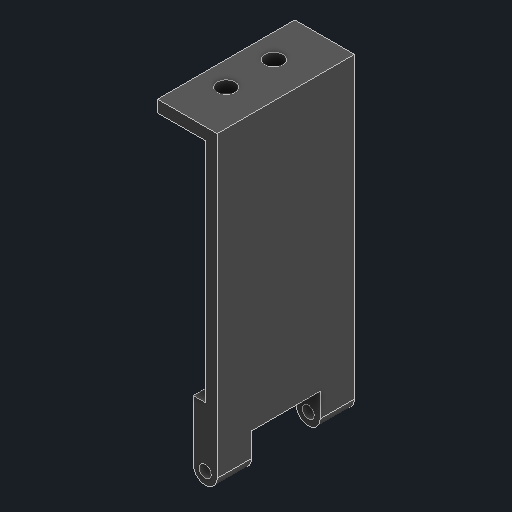
# Autodesk Inventor part: rudder_base
Saved by Autodesk Inventor 2024 (Build 280153000, 153)
## iProperties
Created: 2022-03-30
Part Number: rudder_base
Material: Generic
Document SubType Name: Modeling
Designer: kardo
Density: 1 g/cm^3
Appearance: Dark Plastic
Author: kardo
Autodesk Inventor part; units mm, degrees
ref_plane "YZ Plane" through (0, 0, 0) normal (1, 0, 0) x (0, 1, 0)
ref_plane "XZ Plane" through (0, 0, 0) normal (0, 1, 0) x (-1, 0, 0)
ref_plane "XY Plane" through (0, 0, 0) normal (0, 0, 1) x (1, 0, 0)
derived "parameters_powertrain.ipt"
sketch "sk_base" plane through (0, 0, 0) normal (0, 1, 0) x (-1, 0, 0)
  line L0 (16.1, 0) -> (-16.1, 0) construction
  line L1 (0, -4.6) -> (0, 27.6) construction
  line L2 (0, 23) -> (0, 15.5) construction
  line L3 (0, 7.5) -> (0, 0) construction
  dimension "d13" = 8
  dimension "d36" = 23
  constraints: 4 end point, 3 point on line, 1 collinear
  measures "d13" distance of L3.start L2.end
  measures "d36" distance from line of L0 L2.start
sketch "sk_length" plane through (0, 0, 0) normal (0, 0, 1) x (1, 0, 0)
  line L0 (0, -62.4) -> (0, 10.4) construction
  line L1 (-6, 0) -> (8, 0) construction
  arc A0 (2, -50) -> (6, -50) centre (4, -50) ccw
  line L2 (2, -50) -> (2, -40)
  line L3 (2, -40) -> (4, -40)
  line L4 (4, -40) -> (4, -2)
  line L5 (4, -2) -> (-4, -2)
  line L6 (-4, -2) -> (-4, 0)
  line L7 (-4, 0) -> (6, 0)
  line L8 (6, 0) -> (6, -50)
  point P0 (0, 0)
  dimension "d2" = 50
  dimension "d9" = 2
  dimension "d10" = 4
  dimension "d32" = 4
  dimension "d33" = 10
  dimension "d35" = 4
  constraints: 15 end point, 6 parallel, 3 point on line, 2 point on circle, 2 tangent, 1 centre point, 1 coincident
  measures "d2" distance from line of L1 A0.centre
  measures "d9" distance between parallel lines of L1 L5
  measures "d10" distance between parallel lines of L0 L6
  measures "d32" distance from line of L0 point (4, -50)
  measures "d33" distance of L2.start L2.end
  measures "d35" diameter of A0
extrude "extrude" add sketch "sk_length" along normal up to surface (23 mm away)
hole "drill_base" at (0, 0, 7.5) at (0, 0, 15.5) direction (0, -1, 0) diameter 3 depth 2 tip angle 118
sketch "sk_remove_fin_attach" plane through (2, -50, 0) normal (-1, 0, 0) x (0, 0, 1)
  line L0 (0, 10) -> (23, 10) projected
  line L1 (0, -2) -> (23, -2) projected
  line L2 (0, -2) -> (0, 0) projected
  line L3 (0, -2) -> (0, 10)
  line L4 (0, 10) -> (23, 10) projected
  line L5 (17.25, 10) -> (17.25, -2)
  line L6 (5.75, -2) -> (5.75, 10)
  line L7 (23, 0) -> (23, -2) projected
  line L8 (23, -2) -> (11.5, 10) construction
  line L9 (11.5, 10) -> (0, -2) construction
  line L10 (17.25, 4) -> (5.75, 4)
  point P0 (0, 50)
  constraints: 12 end point, 5 midpoint, 4 point on line, 2 perpendicular
extrude "remove_fin_attach" cut sketch "sk_remove_fin_attach" along normal through all both and the other way through all contours L10 L5 L1 L6
hole "drill_fin" at (4, -50, 0) direction (0, 0, 1) diameter 2 end through all both
equation "\"d13\" = rudder_hole_2_up"
equation "\"d36\" = rudder_body_height"
equation "\"d2\" = rudder_rod_joint_back"
equation "\"d32\" = rudder_axis_location"
equation "\"rudder_hole_2_up\" = 8"
equation "\"rudder_body_height\" = 23"
equation "\"rudder_rod_joint_back\" = 50"
equation "\"rudder_axis_location\" = 4"
body "Solid1"
